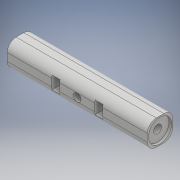
# Autodesk Inventor part: Pieza2
Saved by Autodesk Inventor 2019 (Build 230136000, 136)
## iProperties
Part Number: Pieza2
Material: Genérico
Document SubType Name: Modeling
Designer: beta3
Density: 1 g/cm^3
Appearance: Valor por defecto
Author: beta3
Autodesk Inventor part; units mm, degrees
ref_plane "YZ Plane" through (0, 0, 0) normal (1, 0, 0) x (0, 1, 0)
ref_plane "XZ Plane" through (0, 0, 0) normal (0, 1, 0) x (-1, 0, 0)
ref_plane "XY Plane" through (0, 0, 0) normal (0, 0, 1) x (1, 0, 0)
sketch "Boceto1" plane through (0, 0, 0) normal (0, 1, 0) x (-1, 0, 0)
  line L0 (0, 10) -> (110, 10)
  line L1 (110, 10) -> (110, -10)
  line L2 (110, -10) -> (0, -10)
  line L3 (0, -10) -> (0, 10)
  line L4 (0, 0) -> (110, 0) construction
  line L5 (68.8, -5) -> (75, -5)
  line L6 (75, -5) -> (75, 5)
  line L7 (75, 5) -> (68.8, 5)
  line L8 (68.8, 5) -> (68.8, -5)
  line L9 (71.9, -5) -> (71.9, -10) construction
  line L10 (71.9, 5) -> (71.9, 10) construction
  line L11 (55, -10) -> (55, 10) construction
  line L12 (41.2, -5) -> (35, -5)
  line L13 (35, -5) -> (35, 5)
  line L14 (35, 5) -> (41.2, 5)
  line L15 (41.2, 5) -> (41.2, -5)
  line L16 (58.6062, -3.6062) -> (51.3938, -3.6062) construction
  line L17 (51.3938, -3.6062) -> (51.3938, 3.6062) construction
  line L18 (51.3938, 3.6062) -> (58.6062, 3.6062) construction
  line L19 (58.6062, 3.6062) -> (58.6062, -3.6062) construction
  circle A0 centre (55, 0) radius 4 construction
  circle A1 centre (55, 0) radius 3.05
  circle A2 centre (55, 0) radius 5.1 construction
  dimension "d28" = 10.2
  dimension "d6" = 110
  dimension "d10" = 10
  dimension "d12" = 5
  dimension "d13" = 20
  dimension "d16" = 6.2
  dimension "d18" = 8
  dimension "d19" = 35
  dimension "d27" = 6.1
  constraints: 40 end point, 8 parallel, 7 midpoint, 7 symmetric about line, 6 perpendicular, 4 horizontal, 3 point on line, 2 centre point, 2 coincident, 2 equal length, 3 other
  measures "d6" distance of L1.end L2.end
  measures "d10" distance of L7.end L5.start
  measures "d12" distance between parallel lines of L2 L5
  measures "d13" distance of L0.end L1.end
  measures "d16" distance of L6.end L7.end
  measures "d18" diameter of A0
  measures "d19" distance between parallel lines of L1 L6
  measures "d27" diameter of A1
extrude "Extrusión1" add sketch "Boceto1" along normal blind 20
sketch "Boceto3" plane through (-110, 0, -10) normal (-1, 0, 0) x (0, 0, 1)
  circle A0 centre (10, 10) radius 3.15
  line L0 (20, 20) -> (0, 20) construction
  line L1 (0, 20) -> (20, 0) construction
  line L2 (0, 0) -> (20, 0) construction
  line L3 (20, 20) -> (0, 0) construction
  point P0 (10, 0)
  dimension "d4" = 6.3
  constraints: 4 end point, 1 centre point, 1 coincident, 1 midpoint
  measures "d4" diameter of A0
extrude "Extrusión2" cut sketch "Boceto3" against normal up to next
sketch "Boceto5" plane through (-110, 0, -10) normal (-1, 0, 0) x (0, 0, 1)
  circle A0 centre (10, 10) radius 3.15 projected
  circle A1 centre (10, 10) radius 9.1
  point P0 (10, 0)
  dimension "d8" = 18.2
  constraints: 1 centre point, 1 coincident
  measures "d8" diameter of A1
extrude "Extrusión3" cut sketch "Boceto5" against normal blind 2
sketch "Boceto6" plane through (0, 0, 10) normal (1, 0, 0) x (0, 0, -1)
  circle A0 centre (10, 10) radius 3.15 projected
  circle A1 centre (10, 10) radius 9.1 projected
  point P0 (10, 0)
extrude "Extrusión4" cut sketch "Boceto6" against normal up to next contours A0
sketch "Boceto7" plane through (0, 0, 10) normal (1, 0, 0) x (0, 0, -1)
  circle A0 centre (10, 10) radius 9.1 projected
  point P0 (10, 0)
extrude "Extrusión5" cut sketch "Boceto7" against normal blind 2
fillet "Empalme1" radius 7 4 edges at (-55, 0, 10) (-55, 0, -10) (-55, 20, -10) (-55, 20, 10)
